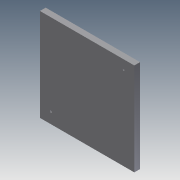
# Autodesk Inventor part: h base
Saved by Autodesk Inventor 2011 (Build 150239000, 239)
## iProperties
Created: 2011-12-04
Part Number: h base
Document SubType Name: Modeling
Designer: Matthew
Density: 1 g/cm^3
Author: Matthew
Autodesk Inventor part; units mm, degrees
ref_plane "YZ Plane" through (0, 0, 0) normal (1, 0, 0) x (0, 1, 0)
ref_plane "XZ Plane" through (0, 0, 0) normal (0, 1, 0) x (-1, 0, 0)
ref_plane "XY Plane" through (0, 0, 0) normal (0, 0, 1) x (1, 0, 0)
sketch "Sketch1" plane through (0, 0, 0) normal (0, 0, 1) x (1, 0, 0)
  line L0 (-22.6981, 19.3174) -> (27.3019, 19.3174)
  line L1 (27.3019, 19.3174) -> (27.3019, -30.6826)
  line L2 (27.3019, -30.6826) -> (-22.6981, -30.6826)
  line L3 (-22.6981, -30.6826) -> (-22.6981, 19.3174)
  point P0 (0, 0)
  dimension "d0" = 50
  dimension "d1" = 50
  constraints: 8 end point, 2 parallel, 1 horizontal, 1 perpendicular
  measures "d0" distance of L1.end L2.end
  measures "d1" distance of L0.end L1.end
extrude "Extrusion1" add sketch "Sketch1" along normal blind 3.175
sketch "Sketch2" plane through (27.3019, -30.6826, 0) normal (1, 0, 0) x (0, 0, -1)
  line L0 (-3.175, 50) -> (-3.175, 0) projected
  line L1 (0, 0) -> (-3.175, 0) projected
  line L2 (0, 50) -> (0, 0) projected
  line L3 (0, 50) -> (-3.175, 50) projected
  point P0 (0, 30.6826)
extrude "Extrusion2" add sketch "Sketch2" along normal blind 9.525
sketch "Sketch3" plane through (0, 0, 3.175) normal (0, 0, 1) x (1, 0, 0)
  line L0 (-22.6981, -30.6826) -> (-22.6981, 19.3174) projected
  line L1 (36.8269, -30.6826) -> (-22.6981, -30.6826) projected
  line L2 (-22.6981, 19.3174) -> (-19.5231, 19.3174)
  line L3 (-19.5231, 19.3174) -> (-19.5231, 4.3174)
  line L4 (-19.5231, 4.3174) -> (-22.6981, 4.3174)
  line L5 (-22.6981, 4.3174) -> (-22.6981, 19.3174)
  line L6 (36.8269, 19.3174) -> (33.6519, 19.3174)
  line L7 (33.6519, 19.3174) -> (33.6519, 4.3174)
  line L8 (33.6519, 4.3174) -> (36.8269, 4.3174)
  line L9 (36.8269, 4.3174) -> (36.8269, 19.3174)
  line L10 (36.8269, -30.6826) -> (33.6519, -30.6826)
  line L11 (33.6519, -30.6826) -> (33.6519, -15.6826)
  line L12 (33.6519, -15.6826) -> (36.8269, -15.6826)
  line L13 (36.8269, -15.6826) -> (36.8269, -30.6826)
  line L14 (-22.6981, -15.6826) -> (-19.5231, -15.6826)
  line L15 (-19.5231, -15.6826) -> (-19.5231, -30.6826)
  line L16 (-19.5231, -30.6826) -> (-22.6981, -30.6826)
  line L17 (-22.6981, -30.6826) -> (-22.6981, -15.6826)
  point P0 (0, 0)
  dimension "d6" = 3.175
  dimension "d7" = 15
  dimension "d8" = 3.175
  dimension "d9" = 15
  constraints: 32 end point, 8 parallel, 4 horizontal, 4 perpendicular, 2 point on line
  measures "d6" distance of L3.end L4.end
  measures "d7" distance of L2.end L3.end
  measures "d8" distance of L8.end L7.end
  measures "d9" distance of L10.end L11.end
extrude "Extrusion3" cut sketch "Sketch3" against normal blind 9.525
sketch "Sketch4" plane through (0, 0, 0) normal (0, 0, -1) x (-1, 0, 0)
  line L0 (-33.6519, -30.6826) -> (19.5231, -30.6826) projected
  line L1 (19.5231, 19.3174) -> (-33.6519, 19.3174) projected
  line L2 (-7.0644, 19.3174) -> (-27.0644, 19.3174)
  line L3 (-27.0644, 19.3174) -> (-27.0644, 14.3174)
  line L4 (-7.0644, -30.6826) -> (12.9356, -30.6826)
  line L5 (12.9356, -30.6826) -> (12.9356, -25.6826)
  circle A0 centre (-27.0644, 14.3174) radius 0.5
  circle A1 centre (12.9356, -25.6826) radius 0.5
  point P0 (0, 0)
  dimension "d12" = 20
  dimension "d13" = 5
  dimension "d14" = 20
  dimension "d15" = 5
  dimension "d16" = 1
  dimension "d17" = 1
  constraints: 8 end point, 2 centre point, 2 coincident, 2 midpoint, 2 perpendicular, 2 point on line
  measures "d12" distance of L2.start L2.end
  measures "d13" distance of L2.end L3.end
  measures "d14" distance of L4.start L4.end
  measures "d15" distance of L4.end L5.end
  measures "d16" diameter of A0
  measures "d17" diameter of A1
extrude "Extrusion4" cut sketch "Sketch4" against normal blind 25.4
sketch "Sketch5" plane through (0, 0, 0) normal (0, 0, -1) x (-1, 0, 0)
  line L0 (-33.6519, 4.3174) -> (-36.8269, 4.3174) projected
  line L1 (-36.8269, 4.3174) -> (-36.8269, -15.6826) projected
  line L2 (-36.8269, -15.6826) -> (-33.6519, -15.6826) projected
  line L3 (-33.6519, -15.6826) -> (-33.6519, -30.6826) projected
  line L4 (-33.6519, -30.6826) -> (19.5231, -30.6826) projected
  line L5 (19.5231, -30.6826) -> (19.5231, -15.6826) projected
  line L6 (19.5231, -15.6826) -> (22.6981, -15.6826) projected
  line L7 (22.6981, -15.6826) -> (22.6981, 4.3174) projected
  line L8 (22.6981, 4.3174) -> (19.5231, 4.3174) projected
  line L9 (19.5231, 4.3174) -> (19.5231, 19.3174) projected
  line L10 (19.5231, 19.3174) -> (-33.6519, 19.3174) projected
  line L11 (-33.6519, 19.3174) -> (-33.6519, 4.3174) projected
  line L12 (19.5231, -30.6826) -> (17.9356, -30.6826)
  line L13 (17.9356, -30.6826) -> (17.9356, 19.3174)
  line L14 (-33.6519, 19.3174) -> (-32.0644, 19.3174)
  line L15 (-32.0644, 19.3174) -> (-32.0644, -30.6826)
  point P0 (0, 0)
  dimension "d20" = 1.5875
  dimension "d21" = 1.5875
  constraints: 8 end point, 4 point on line, 2 perpendicular
  measures "d20" distance of L4.end L12.end
  measures "d21" distance of L10.end L14.end
extrude "Extrusion5" cut sketch "Sketch5" against normal blind 25.4 contours L11 L10 L15 L4 L3 L2 L1 L0 | L10 L9 L8 L7 L6 L5 L4 L13
sketch "Sketch6" plane through (-17.9356, -30.6826, 0) normal (0, -1, 0) x (1, 0, 0)
  line L0 (0, 3.175) -> (0, 0) projected
  line L1 (50, 0) -> (0, 0) projected
  line L2 (50, 0) -> (50, 3.175) projected
  line L3 (50, 3.175) -> (0, 3.175) projected
  point P0 (17.9356, 0)
extrude "Extrusion6" add sketch "Sketch6" along normal blind 3.175
sketch "Sketch7" plane through (-17.9356, 19.3174, 0) normal (-1, 0, 0) x (0, 0, 1)
  line L0 (3.175, 0) -> (3.175, -53.175) projected
  line L1 (0, 0) -> (3.175, 0) projected
  line L2 (0, 0) -> (0, -53.175) projected
  line L3 (0, -53.175) -> (3.175, -53.175) projected
  point P0 (0, -19.3174)
extrude "Extrusion7" add sketch "Sketch7" along normal blind 1.27
sketch "Sketch8" plane through (32.0644, 19.3174, 3.175) normal (1, 0, 0) x (0, 0, -1)
  line L0 (0, -53.175) -> (0, 0) projected
  line L1 (0, -53.175) -> (3.175, -53.175) projected
  line L2 (3.175, 0) -> (3.175, -53.175) projected
  line L3 (0, 0) -> (3.175, 0) projected
  point P0 (3.175, -19.3174)
extrude "Extrusion8" add sketch "Sketch8" along normal blind 1.27
sketch "Sketch9" plane through (-17.9356, -33.8576, 0) normal (0, -1, 0) x (1, 0, 0)
  line L0 (-1.27, 3.175) -> (51.27, 3.175) projected
  line L1 (-1.27, 3.175) -> (-1.27, 0) projected
  line L2 (51.27, 0) -> (-1.27, 0) projected
  line L3 (51.27, 0) -> (51.27, 3.175) projected
  point P0 (17.9356, 0)
extrude "Extrusion9" cut sketch "Sketch9" against normal blind 3.175
sketch "Sketch10" plane through (-17.9356, -30.6826, 0) normal (0, -1, 0) x (1, 0, 0)
  line L0 (-1.27, 0) -> (-1.27, 3.175) projected
  line L1 (51.27, 0) -> (-1.27, 0) projected
  line L2 (51.27, 3.175) -> (51.27, 0) projected
  line L3 (-1.27, 3.175) -> (51.27, 3.175) projected
  point P0 (17.9356, 0)
extrude "Extrusion10" add sketch "Sketch10" along normal blind 1.27
sketch "Sketch11" plane through (33.3344, 19.3174, 3.175) normal (1, 0, 0) x (0, 0, -1)
  line L0 (3.175, 0) -> (3.175, -51.27) projected
  line L1 (0, 0) -> (3.175, 0) projected
  line L2 (0, -51.27) -> (0, 0) projected
  line L3 (0, -51.27) -> (3.175, -51.27) projected
  point P0 (3.175, -19.3174)
extrude "Extrusion11" cut sketch "Sketch11" against normal blind 1.27
sketch "Sketch12" plane through (-17.9356, -31.9526, 0) normal (0, -1, 0) x (1, 0, 0)
  line L0 (50, 0) -> (50, 3.175) projected
  line L1 (-1.27, 3.175) -> (50, 3.175) projected
  line L2 (-1.27, 0) -> (-1.27, 3.175) projected
  line L3 (50, 0) -> (-1.27, 0) projected
  point P0 (17.9356, 0)
extrude "Extrusion12" cut sketch "Sketch12" against normal blind 1.27
sketch "Sketch13" plane through (-19.2056, 19.3174, 0) normal (-1, 0, 0) x (0, 0, 1)
  line L0 (0, -50) -> (3.175, -50) projected
  line L1 (3.175, 0) -> (3.175, -50) projected
  line L2 (0, 0) -> (3.175, 0) projected
  line L3 (0, -50) -> (0, 0) projected
  point P0 (0, -19.3174)
extrude "Extrusion13" cut sketch "Sketch13" against normal blind 1.27
sketch "Sketch14" plane through (-17.9356, -30.6826, 0) normal (0, -1, 0) x (1, 0, 0)
  line L0 (0, 3.175) -> (0, 0) projected
  line L1 (50, 0) -> (0, 0) projected
  line L2 (50, 3.175) -> (50, 0) projected
  line L3 (0, 3.175) -> (50, 3.175) projected
  point P0 (17.9356, 0)
extrude "Extrusion14" add sketch "Sketch14" along normal blind 1
sketch "Sketch15" plane through (-17.9356, 19.3174, 0) normal (-1, 0, 0) x (0, 0, 1)
  line L0 (3.175, 0) -> (3.175, -51) projected
  line L1 (0, 0) -> (3.175, 0) projected
  line L2 (0, 0) -> (0, -51) projected
  line L3 (0, -51) -> (3.175, -51) projected
  point P0 (0, -19.3174)
extrude "Extrusion15" add sketch "Sketch15" along normal blind 1
sketch "Sketch16" plane through (32.0644, 19.3174, 3.175) normal (1, 0, 0) x (0, 0, -1)
  line L0 (3.175, 0) -> (3.175, -51) projected
  line L1 (0, 0) -> (3.175, 0) projected
  line L2 (0, -51) -> (0, 0) projected
  line L3 (0, -51) -> (3.175, -51) projected
  point P0 (3.175, -19.3174)
extrude "Extrusion16" add sketch "Sketch16" along normal blind 1
sketch "Sketch17" plane through (33.0644, 19.3174, 3.175) normal (1, 0, 0) x (0, 0, -1)
  line L0 (3.175, -51) -> (0, -51) projected
  line L1 (3.175, 0) -> (3.175, -51) projected
  line L2 (0, 0) -> (3.175, 0) projected
  line L3 (0, -51) -> (0, 0) projected
  point P0 (3.175, -19.3174)
extrude "Extrusion17" add sketch "Sketch17" along normal blind 2
sketch "Sketch18" plane through (-18.9356, 19.3174, 0) normal (-1, 0, 0) x (0, 0, 1)
  line L0 (3.175, -51) -> (0, -51) projected
  line L1 (3.175, 0) -> (3.175, -51) projected
  line L2 (0, 0) -> (3.175, 0) projected
  line L3 (0, -51) -> (0, 0) projected
  point P0 (0, -19.3174)
extrude "Extrusion18" add sketch "Sketch18" along normal blind 2
body "Solid1"
